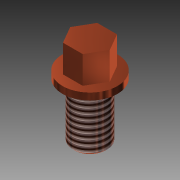
# Autodesk Inventor part: 装填斗罩螺丝
Saved by Autodesk Inventor 2015 (Build 190159000, 159)
## iProperties
Created: 2017-05-23
Part Number: 装填斗罩螺丝
Material: 常规
Document SubType Name: Modeling
Designer: Administrator
Density: 1 g/cm^3
Appearance: 铜 - 抛光
Author: Administrator
Autodesk Inventor part; units mm, degrees
ref_plane "YZ Plane" through (0, 0, 0) normal (1, 0, 0) x (0, 1, 0)
ref_plane "XZ Plane" through (0, 0, 0) normal (0, 1, 0) x (-1, 0, 0)
ref_plane "XY Plane" through (0, 0, 0) normal (0, 0, 1) x (1, 0, 0)
sketch "草图1" plane through (0, 0, 0) normal (0, 0, 1) x (1, 0, 0)
  circle A0 centre (0, 0) radius 4
  dimension "d0" = 8
  constraints: 1 centre point, 1 coincident
  measures "d0" diameter of A0
extrude "拉伸1" add sketch "草图1" along normal blind 1
sketch "草图2" plane through (0, 0, 1) normal (0, 0, 1) x (1, 0, 0)
  line L0 (1.4434, -2.5) -> (-1.4434, -2.5)
  line L1 (-1.4434, -2.5) -> (-2.8868, 0)
  line L2 (-2.8868, 0) -> (-1.4434, 2.5)
  line L3 (-1.4434, 2.5) -> (1.4434, 2.5)
  line L4 (1.4434, 2.5) -> (2.8868, 0)
  line L5 (2.8868, 0) -> (1.4434, -2.5)
  line L6 (0, 0) -> (0, 2.5)
  dimension "d3" = 5
  constraints: 14 end point, 1 coincident, 1 midpoint, 1 vertical, 13 other
  measures "d3" distance between parallel lines of L0 L3
extrude "拉伸2" add sketch "草图2" along normal blind 4
sketch "草图3" plane through (0, 0, 0) normal (0, 0, -1) x (-1, 0, 0)
  circle A0 centre (0, 0) radius 2.5
  dimension "d6" = 5
  constraints: 1 centre point, 1 coincident
  measures "d6" diameter of A0
extrude "拉伸3" add sketch "草图3" along normal blind 8
thread "螺纹1" size "M5x0.8" class "6g" standard "ANSI Metric M Profile" full length
chamfer "倒角1" distance 0.25 angle 45 1 edges at (2.5, 0, -8)
